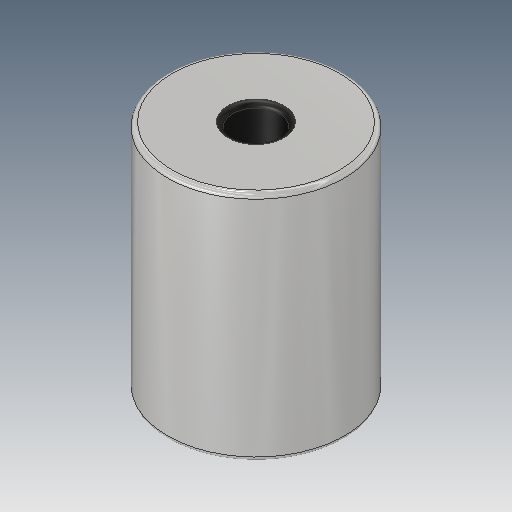
# Autodesk Inventor part: Flx_Al_Coupling(5_8mm)
Saved by Autodesk Inventor 2020 (Build 240168000, 168)
## iProperties
Created: 2018-04-20
Part Number: Flx_Al_Coupling(5_8mm)
Material: Generic
Document SubType Name: Modeling
Designer: PC  USER
Density: 1 g/cm^3
Appearance: Default
Author: PC  USER
Autodesk Inventor part; units mm, degrees
ref_plane "YZ Plane" through (0, 0, 0) normal (1, 0, 0) x (0, 1, 0)
ref_plane "XZ Plane" through (0, 0, 0) normal (0, 1, 0) x (-1, 0, 0)
ref_plane "XY Plane" through (0, 0, 0) normal (0, 0, 1) x (1, 0, 0)
sketch "Sketch1" plane through (0, 0, 0) normal (0, 1, 0) x (-1, 0, 0)
  circle A0 centre (0, 0) radius 9.5
  dimension "d0" = 19
  constraints: 1 centre point, 1 coincident
  measures "d0" diameter of A0
extrude "Extrusion1" add sketch "Sketch1" along normal mid plane 25
sketch "Sketch2" plane through (0, 0, 0) normal (0, 1, 0) x (-1, 0, 0)
  circle A0 centre (0, 0) radius 4
  circle A1 centre (0, 0) radius 2.5
  dimension "d3" = 8
  dimension "d4" = 5
  constraints: 2 centre point, 2 coincident
  measures "d3" diameter of A0
  measures "d4" diameter of A1
extrude "Extrusion2" cut sketch "Sketch2" against normal blind 25 contours A0 | A1
extrude "Extrusion3" cut sketch "Sketch2" along normal blind 25 contours A1
fillet "Fillet1" radius 0.5 4 edges at (9.5, 12.5, 0) (9.5, -12.5, 0) (2.5, 12.5, 0) (4, -12.5, 0)
body "Solid1"
